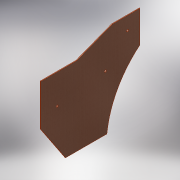
# Autodesk Inventor part: end_plate
Saved by Autodesk Inventor 2018.2 (Build 222227000, 227)
## iProperties
Created: 2017-10-22
Part Number: end_plate
Material: 木材 (オーク)
Document SubType Name: Modeling
Designer: ku_sk
Density: 0.76 g/cm^3
Appearance: ホワイト オーク材 - ナチュラル 標準の光沢
Mass: 1327.49 g
Surface Area: 7114.2 cm^2
Volume: 1746.69 cm^3
Author: ku_sk
Autodesk Inventor part; units mm, degrees
ref_plane "YZ Plane" through (0, 0, 0) normal (1, 0, 0) x (0, 1, 0)
ref_plane "XZ Plane" through (0, 0, 0) normal (0, 1, 0) x (-1, 0, 0)
ref_plane "XY Plane" through (0, 0, 0) normal (0, 0, 1) x (1, 0, 0)
sketch "スケッチ1" plane through (0, 0, 0) normal (1, 0, 0) x (0, 1, 0)
  line L0 (-670, 240) -> (-670, 540)
  line L1 (-670, 540) -> (-400, 720)
  line L2 (-400, 720) -> (-100, 720)
  line L3 (0, 200) -> (0, 0)
  line L4 (0, 0) -> (-230, 0)
  arc A0 (-230, 0) -> (-670, 240) centre (-746.431, -423.4569) ccw
  line L5 (0, 200) -> (-100, 460)
  line L6 (-100, 720) -> (-100, 460)
  point P0 (-200, 720)
  dimension "d0" = 720
  dimension "d1" = 300
  dimension "d2" = 180
  dimension "d3" = 270
  dimension "d4" = 200
  dimension "d5" = 670
  dimension "d6" = 230
  dimension "d75" = 200
  dimension "d76" = 300
  constraints: 14 end point, 3 perpendicular, 2 point on circle, 2 point on line, 1 centre point, 1 coincident, 1 horizontal, 1 parallel
  measures "d0" distance between parallel lines of L4 L2
  measures "d1" distance of L0.start L0.end
  measures "d2" distance from line of L0.end L2
  measures "d3" distance from line of L1.end L0
  measures "d4" distance of L3.start L3.end
  measures "d5" distance between parallel lines of L0 L3
  measures "d6" distance of L3.end L4.end
  measures "d75" distance of L1.end point (-200, 720)
  measures "d76" distance from line of L1.end L6
extrude "押し出し1" add sketch "スケッチ1" along normal blind 5
sketch "スケッチ8" plane through (5, 0, 0) normal (1, 0, 0) x (0, 0, -1)
  circle A0 centre (-600, -315) radius 7.5
  circle A1 centre (-300, -285) radius 7.5
  line L0 (0, 0) -> (-200, 0) projected
  line L1 (0, -230) -> (0, 0) projected
  dimension "d63" = 300
  dimension "d64" = 30
  dimension "d65" = 15
  dimension "d66" = 15
  dimension "d77" = 315
  dimension "d78" = 600
  constraints: 2 centre point
  measures "d63" horizontal distance of A1.centre A0.centre
  measures "d64" vertical distance of A1.centre A0.centre
  measures "d65" diameter of A0
  measures "d66" diameter of A1
  measures "d77" distance from line of L0 A0.centre
  measures "d78" distance from line of L1 A0.centre
extrude "押し出し8" cut sketch "スケッチ8" against normal through all
sketch "スケッチ9" plane through (5, 0, 0) normal (1, 0, 0) x (0, 0, -1)
  circle A0 centre (-90, -95) radius 7.5644
  point P0 (0, 0)
  dimension "d71" = 90
  dimension "d72" = 95
  constraints: 1 centre point
  measures "d71" horizontal distance of point (0, 0) A0.centre
  measures "d72" vertical distance of point (0, 0) A0.centre
extrude "押し出し9" cut sketch "スケッチ9" against normal through all
